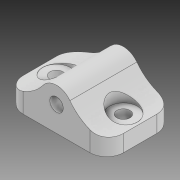
# Autodesk Inventor part: 254 Billet Thrust Block
Saved by Autodesk Inventor 2021 (Build 250183000, 183)
## iProperties
Created: 2021-03-21
Part Number: 254 Billet Thrust Block
Material: Generic
Document SubType Name: Modeling
Density: 1 g/cm^3
Appearance: Default
Autodesk Inventor part; units mm, degrees
ref_plane "YZ Plane" through (0, 0, 0) normal (1, 0, 0) x (0, 1, 0)
ref_plane "XZ Plane" through (0, 0, 0) normal (0, 1, 0) x (-1, 0, 0)
sketch "Sketch1" plane through (0, 0, 0) normal (0, 0, 1) x (1, 0, 0)
  circle A0 centre (0, 0) radius 9.525 construction
  circle A1 centre (0, 0) radius 2.5527
  arc A2 (5.08, 3.81) -> (-5.08, 3.81) centre (0, 0) ccw
  arc A3 (5.08, 3.81) -> (19.05, -3.175) centre (19.05, 14.2875) ccw
  arc A4 (-19.05, -3.175) -> (-5.08, 3.81) centre (-19.05, 14.2875) ccw
  line L0 (-19.05, -9.525) -> (19.05, -9.525)
  line L1 (19.05, -9.525) -> (19.05, -3.175)
  line L2 (-19.05, -9.525) -> (-19.05, -3.175)
  dimension "d0" = 19.05
  dimension "d1" = 5.1054
  dimension "d2" = 12.7
  dimension "d3" = 6.35
  dimension "d4" = 38.1
  constraints: 6 end point, 6 point on circle, 5 centre point, 3 coincident, 3 tangent, 2 line through centre, 1 equal radius, 1 horizontal, 1 horizontal alignment, 1 parallel, 1 perpendicular, 1 vertical
  measures "d0" diameter of A0
  measures "d1" diameter of A1
  measures "d2" diameter of A2
  measures "d3" distance of L0.start L2.end
  measures "d4" distance between parallel lines of L1 L2
extrude "Extrusion1" add sketch "Sketch1" along normal mid plane 25.4
ref_plane "Work Plane1" through (19.05, -3.175, 0) normal (0, 1, 0) x (-1, 0, 0)
sketch "Sketch2" plane through (19.05, -3.175, 0) normal (0, 1, 0) x (-1, 0, 0)
  line L0 (38.1, -12.7) -> (38.1, 12.7) projected
  line L1 (38.1, 0) -> (0, 0)
  line L2 (0, -12.7) -> (0, 12.7) projected
  circle A0 centre (31.75, 0) radius 2.4892
  circle A1 centre (31.75, 0) radius 5.2705
  circle A2 centre (6.35, 0) radius 5.2705
  circle A3 centre (6.35, 0) radius 2.4892
  point P0 (19.05, 0)
  dimension "d7" = 4.9784
  dimension "d8" = 10.541
  dimension "d11" = 360
  dimension "d13" = 25.4
  constraints: 4 centre point, 2 coincident, 2 end point, 2 midpoint, 1 point on line, 9 other
  measures "d7" diameter of A0
  measures "d8" diameter of A1
  measures "d13" distance of A2.centre A0.centre
extrude "Extrusion2" cut sketch "Sketch2" against normal through all contours A0 L1 | L1 A0 | A3 L1 | L1 A3
extrude "Extrusion3" cut sketch "Sketch2" along normal blind 25.4
fillet "Fillet1" radius 6.35 4 edges at (-19.05, -6.35, 12.7) (-19.05, -6.35, -12.7) (19.05, -6.35, 12.7) (19.05, -6.35, -12.7)
body "Solid1"
